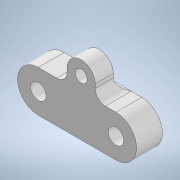
# Autodesk Inventor part: switch_holder
Saved by Autodesk Inventor 2020 (Build 240168000, 168)
## iProperties
Created: 2020-01-22
Part Number: switch_holder
Material: Generic
Document SubType Name: Modeling
Designer: psrobotics
Density: 1 g/cm^3
Appearance: Default
Author: psrobotics
Autodesk Inventor part; units mm, degrees
ref_plane "YZ Plane" through (0, 0, 0) normal (1, 0, 0) x (0, 1, 0)
ref_plane "XZ Plane" through (0, 0, 0) normal (0, 1, 0) x (-1, 0, 0)
ref_plane "XY Plane" through (0, 0, 0) normal (0, 0, 1) x (1, 0, 0)
sketch "Sketch1" plane through (0, 0, 0) normal (0, 0, 1) x (1, 0, 0)
  line L0 (40, 21) -> (41, 20) projected
  line L1 (40, 21) -> (32, 21) projected
  line L2 (32, 21) -> (32, 16) projected
  line L3 (32, 16) -> (35, 16) projected
  arc A0 (36, 15) -> (35, 16) centre (35, 15) ccw projected
  line L4 (36, 15) -> (36, 8) projected
  arc A1 (32, 4) -> (36, 8) centre (32, 8) ccw projected
  line L5 (32, 4) -> (15, 4) projected
  arc A2 (11.4706, 6.1176) -> (15, 4) centre (15, 8) ccw projected
  arc A3 (11.4706, 6.1176) -> (11.4706, -6.1176) centre (0, 0) ccw projected
  arc A4 (15, -4) -> (11.4706, -6.1176) centre (15, -8) ccw projected
  line L6 (15, -4) -> (32, -4) projected
  arc A5 (36, -8) -> (32, -4) centre (32, -8) ccw projected
  line L7 (36, -8) -> (36, -20.0526) projected
  line L8 (36, -20.0526) -> (39.035, -20.6277) projected
  line L9 (41, -19) -> (39.035, -20.6277) projected
  line L10 (41, -19) -> (41, 20) projected
  circle A6 centre (17, 0) radius 1.5 projected
  circle A7 centre (32, 0) radius 1.5 projected
  circle A8 centre (0, 0) radius 8.65 projected
  line L11 (32, 0) -> (17, 0)
  line L12 (32, 0) -> (17, 0) construction
  line L13 (32, 4) -> (17, 4)
  line L14 (17, -4) -> (32, -4)
  arc A9 (32, -4) -> (32, 4) centre (32, 0) ccw
  arc A10 (17, 4) -> (17, -4) centre (17, 0) ccw
  point P0 (0, 0)
  point P1 (24.5, 0)
  dimension "d0" = 7.5
  dimension "d1" = 8
  constraints: 10 end point, 4 point on circle, 4 tangent, 2 centre point, 2 equal length, 2 midpoint, 1 horizontal
  measures "d0" distance of point (24.5, 0) L11.end
  measures "d1" diameter of A10
extrude "Extrusion1" add sketch "Sketch1" along normal blind 3.5 contours L6 A10 L5 A9
thicken "Thicken1" operation add thickness 1.5 both sides no extend neighbours yes toward (0, 0, 1) faces at (22.4427, 2.899, 3.5)
sketch "Sketch2" plane through (17, 4, 5) normal (0, 0, 1) x (1, 0, 0)
  circle A0 centre (8.2825, 2.7175) radius 1.175 projected
  circle A1 centre (8.2825, 2.7175) radius 2.7175
  line L0 (15, 0) -> (0, 0) projected
  line L1 (11, 2.7175) -> (8.2825, 2.7175)
  line L2 (8.2825, 2.7175) -> (5.565, 2.7175)
  line L3 (5.565, 2.7175) -> (5.565, 0)
  line L4 (11, 2.7175) -> (11, 0)
  point P0 (-17, -4)
  constraints: 8 end point, 3 point on line, 2 perpendicular, 2 point on circle, 1 centre point, 1 coincident, 1 horizontal, 1 tangent
extrude "Extrusion2" add sketch "Sketch2" against normal blind 3.5 contours L1 A1 L2 A0 | A0 L2 A1 L1 | L4 L0 A1 | A1 L0 L3
fillet "Fillet1" radius 2 3 edges at (25.2825, 4, 1.5) (22.565, 4, 3.25) (28, 4, 3.25)
body "Solid1"
